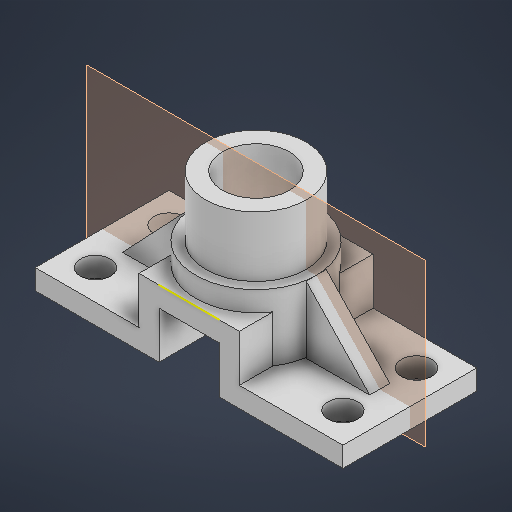
# Autodesk Inventor part: Parte1
Saved by Autodesk Inventor 2026.2 (Build 302298010, 298A)
## iProperties
Created: 2026-03-10
Part Number: Parte1
Material: Generico
Document SubType Name: Modeling
Designer: mahsa
Density: 1 g/cm^3
Appearance: Default
Author: mahsa
Autodesk Inventor part; units mm, degrees
ref_plane "YZ Plane" through (0, 0, 0) normal (1, 0, 0) x (0, 1, 0)
ref_plane "XZ Plane" through (0, 0, 0) normal (0, 1, 0) x (-1, 0, 0)
sketch "Schizzo1" plane through (0, 0, 0) normal (0, 0, 1) x (1, 0, 0)
  line L0 (0, 0) -> (37, 0)
  line L1 (37, 0) -> (37, 6)
  line L2 (37, 6) -> (6, 6)
  line L3 (6, 6) -> (6, 20)
  line L4 (6, 20) -> (-24, 20)
  line L5 (-24, 20) -> (-24, 6)
  line L6 (-24, 6) -> (-55, 6)
  line L7 (-55, 6) -> (-55, 0)
  line L8 (-55, 0) -> (0, 0)
  line L9 (0, 0) -> (-18, 0)
  line L10 (-18, 0) -> (-18, 14)
  line L11 (-18, 14) -> (0, 14)
  line L12 (0, 14) -> (0, 0)
  dimension "d0" = 37
  dimension "d4" = 6
  dimension "d5" = 31
  dimension "d6" = 14
  dimension "d7" = 30
  dimension "d8" = 31
  dimension "d9" = 6
  dimension "d10" = 18
  dimension "d11" = 14
  dimension "d12" = 18
  constraints: 26 end point, 7 perpendicular, 2 horizontal, 1 collinear, 1 point on line, 1 vertical
  measures "d0" distance of L0.start L0.end
  measures "d4" distance of L0.end L1.end
  measures "d5" distance of L1.end L2.end
  measures "d6" distance of L2.end L3.end
  measures "d7" distance of L3.end L4.end
  measures "d8" distance of L5.end L6.end
  measures "d9" distance of L6.end L7.end
  measures "d10" distance of L0.start L9.end
  measures "d11" distance of L9.end L10.end
  measures "d12" distance of L10.end L11.end
extrude "Estrusione1" add sketch "Schizzo1" along normal blind 20 and the other way blind 20 contours L12 L11 L10 L8 L7 L6 L5 L4 L3 L2 L1 L0
sketch "Schizzo2" plane through (6, 6, 20) normal (1, 0, 0) x (0, 0, -1)
  point P0 (20, -6)
sketch "Schizzo3" plane through (6, 6, 20) normal (0, 1, 0) x (1, 0, 0)
  line L0 (31, 40) -> (31, 0) projected
  line L1 (31, 40) -> (31, 31)
  line L2 (31, 31) -> (31, 40)
  line L3 (31, 31) -> (22, 31)
  circle A0 centre (22, 31) radius 4.5
  point P0 (-6, 20)
  dimension "d17" = 9
  dimension "d19" = 9
  dimension "d20" = 9
  constraints: 6 end point, 1 centre point, 1 coincident, 1 collinear, 1 perpendicular, 1 point on line
  measures "d17" distance of L0.start L1.end
  measures "d19" distance of L1.end L3.end
  measures "d20" diameter of A0
extrude "Estrusione2" cut sketch "Schizzo3" against normal blind 6
sketch "Schizzo4" plane through (6, 6, 20) normal (0, 1, 0) x (1, 0, 0)
  circle A0 centre (22, 31) radius 4.5 projected
  line L0 (22, 31) -> (22, 9)
  circle A1 centre (22, 9) radius 4.5
  point P0 (-6, 20)
  dimension "d23" = 22
  dimension "d24" = 9
  constraints: 2 end point, 1 centre point, 1 coincident, 1 vertical
  measures "d23" distance of L0.start L0.end
  measures "d24" diameter of A1
extrude "Estrusione3" cut sketch "Schizzo4" against normal blind 9 contours A1
sketch "Schizzo5" plane through (-55, 6, 20) normal (0, 1, 0) x (1, 0, 0)
  line L0 (0, 40) -> (31, 40) projected
  line L1 (0, 40) -> (0, 31)
  line L2 (0, 40) -> (0, 0) projected
  line L3 (0, 31) -> (9, 31)
  line L4 (9, 31) -> (9, 9)
  circle A0 centre (9, 31) radius 4.5
  circle A1 centre (9, 9) radius 4.5
  point P0 (55, 20)
  dimension "d27" = 9
  dimension "d28" = 9
  dimension "d29" = 22
  dimension "d30" = 9
  dimension "d31" = 9
  constraints: 6 end point, 2 centre point, 2 coincident, 2 perpendicular, 1 point on line
  measures "d27" distance of L0.start L1.end
  measures "d28" distance of L1.end L3.end
  measures "d29" distance of L3.end L4.end
  measures "d30" diameter of A0
  measures "d31" diameter of A1
extrude "Estrusione4" cut sketch "Schizzo5" against normal blind 6
sketch "Schizzo6" plane through (-24, 20, 20) normal (0, 1, 0) x (1, 0, 0)
  line L0 (6, 0) -> (24, 0) projected
  point P0 (24, 20)
ref_plane "Piano di lavoro1" through (-24, 26, 20) normal (0, 1, 0) x (1, 0, 0)
sketch "Schizzo7" plane through (0, 0, -20) normal (0, 0, -1) x (-1, 0, 0)
  point P0 (0, 0)
sketch "Schizzo8" plane through (-24, 20, 20) normal (0, 1, 0) x (1, 0, 0)
  line L0 (0, 40) -> (0, 0) projected
  line L1 (0, 0) -> (-20, 0)
  line L2 (6, 0) -> (24, 0) projected
  line L3 (15, 0) -> (15, 20)
  circle A0 centre (15, 20) radius 18
  point P0 (24, 20)
  dimension "d37" = 20
  dimension "d38" = 20
  dimension "d39" = 36
  constraints: 4 end point, 1 centre point, 1 coincident, 1 collinear, 1 midpoint, 1 vertical
  measures "d37" distance of L0.end L1.end
  measures "d38" distance of L3.start L3.end
  measures "d39" diameter of A0
extrude "Estrusione5" add sketch "Schizzo8" against normal through all
sketch "Schizzo9" plane through (-24, 20, 20) normal (0, 1, 0) x (1, 0, 0)
  arc A0 (0, 29.9499) -> (0, 10.0501) centre (15, 20) ccw projected
  circle A1 centre (15, 20) radius 18
  point P0 (24, 20)
  point P1 (0, 10.0501)
  dimension "d44" = 36
  constraints: 1 centre point, 1 coincident
  measures "d44" diameter of A1
extrude "Estrusione6" add sketch "Schizzo9" along normal blind 6
sketch "Schizzo10" plane through (-24, 26, 20) normal (0, 1, 0) x (1, 0, 0)
  arc A0 (30, 29.9499) -> (0, 29.9499) centre (15, 20) ccw projected
  circle A1 centre (15, 20) radius 10
  circle A2 centre (15, 20) radius 15
  point P0 (24, 20)
  dimension "d47" = 20
  dimension "d48" = 30
  constraints: 2 centre point, 2 coincident
  measures "d47" diameter of A1
  measures "d48" diameter of A2
extrude "Estrusione7" add sketch "Schizzo10" along normal blind 18
sketch "Schizzo12" plane through (0, 0, 0) normal (0, 0, 1) x (1, 0, 0)
  line L0 (-27, 6) -> (-24, 6) projected
  line L1 (-24, 26) -> (-27, 26) projected
  line L2 (-27, 26) -> (-45.9113, 6)
  point P0 (0, 0)
  point P1 (-55, 6)
  point P2 (9, 26)
  constraints: 2 end point
extrude "Nervatura2" add sketch "Schizzo12" along normal mid plane 6 rib yes fills toward (-25.5, 25.95) open curves L1 L2
sketch "Schizzo13" plane through (0, 0, 0) normal (0, 0, 1) x (1, 0, 0)
  line L0 (37, 6) -> (28, 6)
  line L1 (28, 6) -> (9, 26)
  line L2 (9, 26) -> (9, 6)
  line L3 (9, 26) -> (9, 6) projected
  point P0 (0, 0)
  dimension "d66" = 9
  constraints: 6 end point, 2 point on line, 1 horizontal
  measures "d66" distance of L0.start L0.end
extrude "Nervatura3" add sketch "Schizzo13" along normal mid plane 6 rib yes fills toward (32.5, 5.95) open curves L0 L1 L2
equation "\"d25\" = d24"
